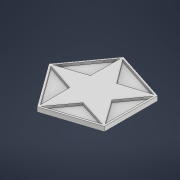
# Autodesk Inventor part: Pieza de practica 1
Saved by Autodesk Inventor 2022 (Build 260153000, 153)
## iProperties
Created: 2022-05-30
Part Number: Pieza de practica 1
Material: Genérico
Document SubType Name: Modeling
Designer: aleon
Density: 1 g/cm^3
Appearance: Valor por defecto
Author: aleon
Autodesk Inventor part; units mm, degrees
ref_plane "YZ Plane" through (0, 0, 0) normal (1, 0, 0) x (0, 1, 0)
ref_plane "XZ Plane" through (0, 0, 0) normal (0, 1, 0) x (-1, 0, 0)
ref_plane "XY Plane" through (0, 0, 0) normal (0, 0, 1) x (1, 0, 0)
sketch "Boceto1" plane through (0, 0, 0) normal (0, 1, 0) x (-1, 0, 0)
  circle A0 centre (0, 0) radius 10
  line L0 (10, 0) -> (3.0902, -9.5106)
  line L1 (3.0902, -9.5106) -> (-8.0902, -5.8779)
  line L2 (-8.0902, -5.8779) -> (-8.0902, 5.8779)
  line L3 (-8.0902, 5.8779) -> (3.0902, 9.5106)
  line L4 (3.0902, 9.5106) -> (10, 0)
  line L5 (-7.6902, -5.5872) -> (2.9374, -9.0403)
  line L6 (2.9374, -9.0403) -> (9.5056, 0)
  line L7 (9.5056, 0) -> (2.9374, 9.0403)
  line L8 (2.9374, 9.0403) -> (-7.6902, 5.5872)
  line L9 (-7.6902, 5.5872) -> (-7.6902, -5.5872)
  dimension "d0" = 20
  dimension "d1" = 0.4
  constraints: 20 end point, 2 coincident, 1 horizontal alignment, 17 other
  measures "d1" distance between parallel lines of L1 L5
extrude "Extrusión1" add sketch "Boceto1" along normal blind 1 contours L0 L1 L2 L3 L4
extrude "Extrusión2" add sketch "Boceto1" along normal blind 0.5 contours L9 L8 L7 L6 L5
sketch "Boceto2" plane through (0, 0.5, 0) normal (0, 1, 0) x (1, 0, 0)
  line L0 (8.0902, -5.8779) -> (8.0902, 5.8779) projected
  line L1 (8.0902, -5.8779) -> (3.9, 0)
  line L2 (3.9, 0) -> (8.0902, 5.8779)
  circle A0 centre (0, 0) radius 10 projected
  line L3 (8.0902, 5.8779) -> (1.2052, 3.7091)
  line L4 (1.2052, 3.7091) -> (-3.0902, 9.5106)
  line L5 (-3.0902, 9.5106) -> (-3.1552, 2.2924)
  line L6 (-3.1552, 2.2924) -> (-10, 0)
  line L7 (-10, 0) -> (-3.1552, -2.2924)
  line L8 (-3.1552, -2.2924) -> (-3.0902, -9.5106)
  line L9 (-3.0902, -9.5106) -> (1.2052, -3.7091)
  line L10 (1.2052, -3.7091) -> (8.0902, -5.8779)
  dimension "d6" = 3.9
  dimension "d9" = 360
  constraints: 20 end point, 26 other
  measures "d6" distance of L1.end point (0, 0)
extrude "Extrusión3" add sketch "Boceto2" along normal blind 0.5 contours L10 L9 L8 L7 L6 L5 L4 L3 L2 L1
